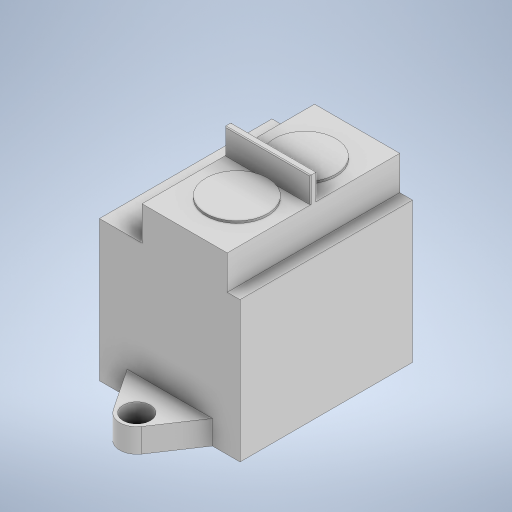
# Autodesk Inventor part: Pieza3-Tarea2
Saved by Autodesk Inventor 2024 (Build 280153000, 153)
## iProperties
Created: 2024-02-22
Part Number: Pieza3-Tarea2
Material: Genérico
Document SubType Name: Modeling
Designer: Diegolap
Density: 1 g/cm^3
Appearance: Valor por defecto
Author: Diegolap
Autodesk Inventor part; units mm, degrees
ref_plane "YZ Plane" through (0, 0, 0) normal (1, 0, 0) x (0, 1, 0)
ref_plane "XZ Plane" through (0, 0, 0) normal (0, 1, 0) x (-1, 0, 0)
ref_plane "XY Plane" through (0, 0, 0) normal (0, 0, 1) x (1, 0, 0)
sketch "Boceto1" plane through (0, 0, 0) normal (0, 0, 1) x (1, 0, 0)
  line L0 (0, 0) -> (33, 0)
  line L1 (33, 0) -> (33, 33)
  line L2 (33, 33) -> (0, 33)
  line L3 (0, 33) -> (0, 0)
  line L4 (10, 33) -> (30, 33)
  line L5 (30, 33) -> (30, 41)
  line L6 (30, 41) -> (10, 41)
  line L7 (10, 41) -> (10, 33)
  point P0 (30, 33)
  dimension "d4" = 33
  dimension "d5" = 33
  dimension "d6" = 41
  dimension "d7" = 3
  dimension "d8" = 10
  constraints: 16 end point, 4 parallel, 2 horizontal, 2 perpendicular, 1 coincident, 1 point on line
  measures "d4" distance of L0.start L0.end
  measures "d5" distance of L2.end L0.start
  measures "d6" distance between parallel lines of L0 L6
  measures "d7" distance from line of L1.end L5
  measures "d8" distance from line of L2.end L7
extrude "Extrusión1" add sketch "Boceto1" along normal blind 40.5
sketch "Boceto2" plane through (10, 41, 0) normal (0, 1, 0) x (1, 0, 0)
  line L0 (20, -21) -> (0, -21)
  line L1 (0, -21) -> (0, -19.5)
  line L2 (0, -19.5) -> (20, -19.5)
  line L3 (20, -19.5) -> (20, -21)
  line L4 (0, 0) -> (0, -40.5) projected
  line L5 (20, 0) -> (20, -40.5) projected
  point P0 (-10, 0)
  point P1 (0, -20.25)
  point P2 (20, -20.25)
  dimension "d11" = 1.5
  constraints: 8 end point, 4 midpoint, 2 parallel, 1 horizontal, 1 perpendicular
  measures "d11" distance of L2.end L0.start
extrude "Extrusión2" add sketch "Boceto2" along normal blind 6
fillet "Empalme1" radius 0.2 6 edges at (10, 44, 21) (20, 47, 21) (30, 44, 21) (10, 44, 19.5) (20, 47, 19.5) (30, 44, 19.5)
sketch "Boceto3" plane through (10, 41, 40.5) normal (0, 1, 0) x (1, 0, 0)
  line L0 (0, 40.5) -> (0, 0) projected
  line L1 (0, 20.25) -> (20, 20.25)
  line L2 (20, 40.5) -> (20, 0) projected
  line L3 (10, 20.25) -> (10, 28.25)
  line L4 (10, 20.25) -> (10, 12.25)
  line L5 (19.8, 19.5) -> (0.2, 19.5) projected
  line L6 (10, 19.5) -> (12.8197, 19.5)
  line L7 (0.2, 21) -> (19.8, 21) projected
  line L8 (10, 21) -> (12.8197, 21)
  circle A0 centre (10, 12.25) radius 7.25
  circle A1 centre (10, 28.25) radius 7.25
  point P0 (-10, 40.5)
  dimension "d15" = 8
  dimension "d16" = 8
  constraints: 10 end point, 5 midpoint, 2 coincident, 2 point on line, 2 vertical, 1 centre point, 1 tangent, 1 vertical alignment, 2 other
  measures "d15" distance of L3.start L3.end
  measures "d16" distance of L3.start L4.end
extrude "Extrusión3" add sketch "Boceto3" along normal blind 0.5
sketch "Boceto4" plane through (0, 0, 0) normal (0, -1, 0) x (1, 0, 0)
  line L0 (0, 0) -> (33, 0) projected
  line L1 (16.5, 0) -> (16.5, 40.5)
  line L2 (0, 40.5) -> (33, 40.5) projected
  line L3 (16.5, 20.25) -> (16.5, 48.25)
  circle A0 centre (16.5, 48.25) radius 3.2
  circle A1 centre (16.5, 48.25) radius 4
  line L4 (16.5, 40.5) -> (6.5, 40.5)
  line L5 (16.5, 40.5) -> (26.5, 40.5)
  line L6 (26.5, 40.5) -> (19.8242, 50.4748)
  line L7 (6.5, 40.5) -> (13.1758, 50.4748)
  line L8 (16.5, 20.25) -> (16.5, -7.75)
  circle A2 centre (16.5, -7.75) radius 3.2
  circle A3 centre (16.5, -7.75) radius 4
  line L9 (6.5, 0) -> (26.5, 0)
  line L10 (6.5, 0) -> (13.1758, -9.9748)
  line L11 (26.5, 0) -> (19.8242, -9.9748)
  dimension "d19" = 28
  dimension "d20" = 6.4
  dimension "d21" = 8
  dimension "d22" = 10
  dimension "d23" = 10
  dimension "d26" = 28
  dimension "d27" = 6.4
  dimension "d28" = 8
  dimension "d29" = 20
  dimension "d30" = 6.5
  constraints: 20 end point, 6 point on line, 5 midpoint, 4 centre point, 4 coincident, 4 point on circle, 4 tangent
  measures "d19" distance of L3.end L3.start
  measures "d20" diameter of A0
  measures "d21" diameter of A1
  measures "d22" distance of point (16.5, 40.5) L4.end
  measures "d23" distance of L5.end point (16.5, 40.5)
  measures "d26" distance of L3.start L8.end
  measures "d27" diameter of A2
  measures "d28" diameter of A3
  measures "d29" distance of L9.start L9.end
  measures "d30" distance of L0.start L9.start
extrude "Extrusión4" add sketch "Boceto4" against normal blind 5.6
equation "\"d4\" = DistA"
equation "\"d5\" = DistC"
equation "\"d6\" = DistB"
equation "\"d9\" = DistEXT"
equation "\"d12\" = DistEXT2"
equation "\"d24\" = DistEXT3"
equation "\"DistA\" = 33"
equation "\"DistB\" = 41"
equation "\"DistEXT\" = 40.5"
equation "\"DistC\" = 33"
equation "\"DistEXT2\" = 6"
equation "\"DistEXT3\" = 5.6"
